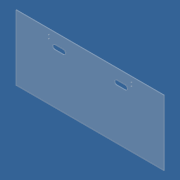
# Autodesk Inventor part: FE-00011
Saved by Autodesk Inventor 2012 (Build 160160000, 160)
## iProperties
Created: 2008-06-02
Part Number: FE-00011
Document SubType Name: Modeling
Designer: mcyr
Density: 1 g/cm^3
Description: Field Plastic "G"
Mass: 3310.59 g
Surface Area: 10660.9 cm^2
Volume: 3310.59 cm^3
Material: Default
Title: FE-00011
Author: mcyr
Autodesk Inventor part; units mm, degrees
ref_plane "YZ Plane" through (0, 0, 0) normal (1, 0, 0) x (0, 1, 0)
ref_plane "XZ Plane" through (0, 0, 0) normal (0, 1, 0) x (-1, 0, 0)
ref_plane "XY Plane" through (0, 0, 0) normal (0, 0, 1) x (1, 0, 0)
sketch "Sketch1" plane through (0, 0, 0) normal (0, 0, 1) x (1, 0, 0)
  line L0 (-130.5517, -4.3675) -> (961.6483, -4.3675)
  line L1 (961.6483, -4.3675) -> (961.6483, 478.2325)
  line L2 (961.6483, 478.2325) -> (-130.5517, 478.2325)
  line L3 (-130.5517, 478.2325) -> (-130.5517, -4.3675)
  arc A0 (155.1983, 398.8575) -> (155.1983, 367.1075) centre (155.1983, 382.9825) ccw
  arc A1 (218.6983, 367.1075) -> (218.6983, 398.8575) centre (218.6983, 382.9825) ccw
  line L4 (155.1983, 398.8575) -> (218.6983, 398.8575)
  line L5 (218.6983, 367.1075) -> (155.1983, 367.1075)
  arc A2 (612.3983, 400.445) -> (612.3983, 368.695) centre (612.3983, 384.57) ccw
  arc A3 (675.8983, 368.695) -> (675.8983, 400.445) centre (675.8983, 384.57) ccw
  line L6 (612.3983, 400.445) -> (675.8983, 400.445)
  line L7 (675.8983, 368.695) -> (612.3983, 368.695)
  circle A4 centre (110.7483, 440.1325) radius 3.175
  circle A5 centre (110.7483, 414.7325) radius 3.175
  circle A6 centre (720.3483, 440.1325) radius 3.175
  circle A7 centre (720.3483, 414.7325) radius 3.175
  dimension "d0" = 1092.2
  dimension "d1" = 482.6
  dimension "d4" = 63.5
  dimension "d5" = 95.25
  dimension "d6" = 285.75
  dimension "d7" = 63.5
  dimension "d9" = 285.75
  dimension "d14" = 38.1
  dimension "d15" = 63.5
  dimension "d16" = 241.3
  dimension "d17" = 241.3
  dimension "d18" = 38.1
  dimension "d19" = 63.5
  dimension "d20" = 850.9
  dimension "d21" = 850.9
  dimension "d24" = 15.875
  constraints: 16 end point, 8 centre point, 8 point on circle, 6 tangent, 2 parallel, 1 horizontal, 1 perpendicular
  measures "d0" distance of L0.start L0.end
  measures "d1" distance of L2.end L0.start
  measures "d4" distance of A1.centre A0.centre
  measures "d5" vertical distance of L2.end A0.centre
  measures "d6" horizontal distance of A0.centre L2.end
  measures "d7" distance of A3.centre A2.centre
  measures "d9" horizontal distance of L1.end A3.centre
  measures "d14" vertical distance of L2.end A4.centre
  measures "d15" distance from line of L2 A5.centre
  measures "d16" distance from line of L3 A4.centre
  measures "d17" distance from line of L3 A5.centre
  measures "d18" distance from line of L2 A6.centre
  measures "d19" distance from line of L2 A7.centre
  measures "d20" horizontal distance of L2.end A6.centre
  measures "d21" horizontal distance of L2.end A7.centre
  measures "d24" radius of A3
extrude "Extrusion1" add sketch "Sketch1" along normal blind 6.35
body "Solid1"
